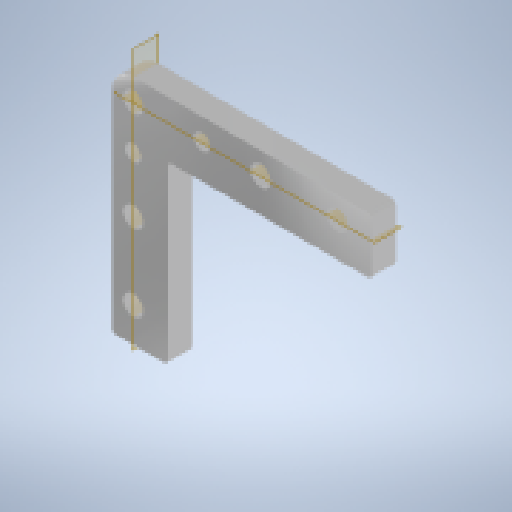
# Autodesk Inventor part: Top Corner Extrusion Plate
Saved by Autodesk Inventor 2024 (Build 280153000, 153)
## iProperties
Created: 2024-08-20
Part Number: Top Corner Extrusion Plate
Material: Aluminum 6061
Document SubType Name: Modeling
Designer: Ishaan
Density: 2.7 g/cm^3
Appearance: Aluminum - Flat
Author: Ishaan
Autodesk Inventor part; units mm, degrees
ref_plane "YZ Plane" through (0, 0, 0) normal (1, 0, 0) x (0, 1, 0)
ref_plane "XZ Plane" through (0, 0, 0) normal (0, 1, 0) x (-1, 0, 0)
ref_plane "XY Plane" through (0, 0, 0) normal (0, 0, 1) x (1, 0, 0)
sketch "Sketch1" plane through (0, 0, 0) normal (0, 0, 1) x (1, 0, 0)
  line L0 (26.675, -23) -> (-26.675, -23) construction
  line L1 (-26.675, -23) -> (-26.675, 23) construction
  line L2 (-26.675, 23) -> (26.675, 23) construction
  line L3 (26.675, 23) -> (26.675, -23) construction
  line L4 (26.675, -23) -> (-26.675, 23) construction
  line L5 (-26.675, -23) -> (26.675, 23) construction
  line L6 (-26.675, -23) -> (-41.325, -23)
  line L7 (-41.325, -23) -> (-41.325, 15)
  line L8 (-41.325, 15) -> (-26.675, 15)
  line L9 (-26.675, 15) -> (-26.675, -23)
  line L10 (26.675, 23) -> (-11.325, 23)
  line L11 (-11.325, 23) -> (-11.325, 37.65)
  line L12 (-11.325, 37.65) -> (26.675, 37.65)
  line L13 (26.675, 37.65) -> (26.675, 23)
  line L14 (-35.675, -23) -> (-35.675, 32) construction
  line L15 (-35.675, 32) -> (26.675, 32) construction
  circle A0 centre (-35.675, 32) radius 5.65 construction
  line L16 (-26.675, 15) -> (-41.325, 15)
  line L17 (-41.325, 15) -> (-41.325, 37.65)
  line L18 (-35.675, 37.65) -> (-26.675, 37.65)
  line L19 (-26.675, 37.65) -> (-26.675, 15)
  line L20 (-11.325, 23) -> (-41.325, 23)
  line L21 (-41.325, 23) -> (-41.325, 32)
  line L22 (-41.325, 37.65) -> (-11.325, 37.65)
  line L23 (-11.325, 37.65) -> (-11.325, 23)
  arc A1 (-35.675, 37.65) -> (-41.325, 32) centre (-35.675, 32) ccw
  point P0 (0, 0)
  point P1 (0, 0)
  point P2 (-26.675, 23)
  point P3 (-41.325, 32)
  point P4 (-35.675, -14)
  point P5 (-35.675, 6)
  point P6 (17.675, 32)
  point P7 (-2.325, 32)
  dimension "d3" = 9
  dimension "d4" = 9
  dimension "d5" = 5.65
  dimension "d6" = 5.65
  dimension "d8" = 8
  dimension "d9" = 15.35
  dimension "d13" = 5.65
  dimension "d14" = 9
  dimension "d15" = 20
  dimension "d16" = 5.65
  dimension "d17" = 9
  dimension "d18" = 20
  dimension "d33" = 9
  dimension "d35" = 9
  constraints: 48 end point, 10 parallel, 8 point on line, 6 perpendicular, 5 horizontal, 4 tangent, 3 coincident, 2 centre point, 2 midpoint, 2 point on circle, 1 collinear, 1 concentric, 1 vertical
  measures "d3" distance between parallel lines of L2 L15
  measures "d4" distance between parallel lines of L14 L1
  measures "d5" distance between parallel lines of L7 L14
  measures "d6" distance between parallel lines of L15 L12
  measures "d8" distance between parallel lines of L16 L20
  measures "d9" distance between parallel lines of L23 L19
  measures "d13" distance from line of L12 point (17.675, 32)
  measures "d14" distance from line of L13 point (17.675, 32)
  measures "d15" distance of point (-2.325, 32) point (17.675, 32)
  measures "d16" distance from line of L7 point (-35.675, -14)
  measures "d17" distance from line of L6 point (-35.675, -14)
  measures "d18" distance of point (-35.675, 6) point (-35.675, -14)
  measures "d33" distance from line of point (-2.325, 32) L11
  measures "d35" distance from line of L8 point (-35.675, 6)
extrude "Extrusion1" add sketch "Sketch1" along normal mid plane 6.35 contours L6 L7 L8 L9 | L8 L17 L20 L19 | L20 L17 A1 L18 L19 | L19 L22 L11 L20 | L11 L12 L13 L10
sketch "Sketch2" plane through (0, 0, 3.175) normal (0, 0, 1) x (1, 0, 0)
  line L0 (-41.325, -23) -> (-26.675, -23) projected
  line L1 (-26.675, -23) -> (-26.675, 23) projected
  line L2 (-26.675, 23) -> (26.675, 23) projected
  line L3 (26.675, 23) -> (26.675, 37.65) projected
  line L4 (26.675, 37.65) -> (-35.675, 37.65) projected
  arc A0 (-35.675, 37.65) -> (-41.325, 32) centre (-35.675, 32) ccw construction
  line L5 (-41.325, 32) -> (-41.325, -23) projected
  line L6 (-25.675, 22) -> (-45.675, 22) construction
  line L7 (-45.675, 22) -> (-45.675, 42) construction
  line L8 (-45.675, 42) -> (-25.675, 42) construction
  line L9 (-25.675, 42) -> (-25.675, 22) construction
  line L10 (-25.675, 22) -> (-45.675, 42) construction
  line L11 (-45.675, 22) -> (-25.675, 42) construction
  point P0 (0, 0)
  dimension "d31" = 20
  dimension "d32" = 20
  constraints: 12 end point, 2 midpoint, 2 parallel, 1 horizontal, 1 perpendicular
  measures "d31" distance of L7.end L8.end
  measures "d32" distance of L6.end L7.end
hole "Hole1" at (-35.675, 6, 0) at (-35.675, -14, 0) at (-2.325, 32, 0) at (17.675, 32, 0) at (-35.675, 32, 0) direction (0, 0, -1) diameter 5.3 end through all both
fillet "Fillet1" radius 1 1 edges at (-26.675, 23, 0)
fillet "Fillet2" radius 1 4 edges at (26.675, 23, 0) (26.675, 37.65, 0) (-26.675, -23, 0) (-41.325, -23, 0)
ref_plane "Work Plane1" through (-2.325, 32, 0) normal (0, 1, 0) x (0, 0, 1)
ref_plane "Work Plane2" through (-35.675, 6, 0) normal (1, 0, 0) x (0, 0, 1)
sketch "Sketch3" plane through (0, 0, 3.175) normal (0, 0, 1) x (1, 0, 0)
  arc A0 (-41.325, -22) -> (-40.325, -23) centre (-40.325, -22) ccw projected
  line L0 (-40.325, -23) -> (-27.675, -23) projected
  arc A1 (-27.675, -23) -> (-26.675, -22) centre (-27.675, -22) ccw projected
  line L1 (-26.675, -22) -> (-26.675, 22) projected
  arc A2 (-25.675, 23) -> (-26.675, 22) centre (-25.675, 22) ccw projected
  line L2 (-25.675, 23) -> (25.675, 23) projected
  arc A3 (25.675, 23) -> (26.675, 24) centre (25.675, 24) ccw projected
  line L3 (26.675, 24) -> (26.675, 36.65) projected
  arc A4 (26.675, 36.65) -> (25.675, 37.65) centre (25.675, 36.65) ccw projected
  line L4 (25.675, 37.65) -> (-35.675, 37.65) projected
  arc A5 (-35.675, 37.65) -> (-41.325, 32) centre (-35.675, 32) ccw projected
  line L5 (-41.325, 32) -> (-41.325, -22) projected
  circle A6 centre (-35.675, 32) radius 2.65 projected
  circle A7 centre (17.675, 32) radius 2.65 projected
  circle A8 centre (-2.325, 32) radius 2.65 projected
  circle A9 centre (-35.675, -14) radius 2.65 projected
  circle A10 centre (-35.675, 6) radius 2.65 projected
  point P0 (0, 0)
  point P1 (-17.675, 32)
  point P2 (-35.675, 20.5)
  dimension "d36" = 11.5
  dimension "d37" = 18
  constraints: 1 horizontal alignment, 1 vertical alignment
  measures "d36" distance of point (-35.675, 20.5) A5.centre
  measures "d37" distance of point (-17.675, 32) A5.centre
hole "Hole2" at (-17.675, 32, 3.175) direction (0, 0, -1) diameter 5.2 end through all
equation "\"d4\" = d3"
equation "\"d6\" = d5"
equation "\"d14\" = d33"
equation "\"d17\" = d35"
equation "\"d18\" = d15"
equation "\"d33\" = d3"
equation "\"d35\" = d4"
body "Solid1"
